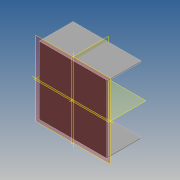
# Autodesk Inventor part: P004_CageDeTest2
Saved by Autodesk Inventor 2020 (Build 240168000, 168)
## iProperties
Created: 2021-09-24
Part Number: P004_CageDeTest2
Material: Générique
Document SubType Name: Modeling
Designer: gabri
Density: 1 g/cm^3
Appearance: Par défaut
Author: gabri
Autodesk Inventor part; units mm, degrees
sketch "Esquisse2" plane through (0, 0, 0) normal (0, 1, 0) x (-1, 0, 0)
  line L0 (1000, 1000) -> (-1000, 1000)
  line L1 (-1000, 1000) -> (-1000, -1000)
  line L2 (-1000, -1000) -> (1000, -1000)
  line L3 (1000, -1000) -> (1000, 1000)
  line L4 (0, -1400) -> (0, 1400) construction
  line L5 (1400, 0) -> (-1400, 0) construction
  point P0 (0, 0)
  dimension "d0" = 2000
  dimension "d1" = 2000
  dimension "d2" = 1000
  dimension "d3" = 1000
  constraints: 8 end point, 2 parallel, 1 horizontal, 1 perpendicular
  measures "d0" distance of L0.end L1.end
  measures "d1" distance of L0.start L0.end
  measures "d2" distance between parallel lines of L4 L1
  measures "d3" distance between parallel lines of L5 L0
extrude "Extrusion1" add sketch "Esquisse2" along normal blind 1000
sketch "Esquisse3" plane through (0, 1000, 0) normal (0, 1, 0) x (1, 0, 0)
  line L0 (-960, -960) -> (960, -960)
  line L1 (960, -960) -> (960, 960)
  line L2 (960, 960) -> (-960, 960)
  line L3 (-960, 960) -> (-960, -960)
  line L4 (1000, 1000) -> (-1000, 1000) construction
  line L5 (-1000, -1000) -> (1000, -1000) construction
  line L6 (-1000, 1000) -> (-1000, -1000) construction
  line L7 (1000, -1000) -> (1000, 1000) construction
  point P0 (0, 0)
  dimension "d6" = 40
  dimension "d7" = 40
  dimension "d8" = 40
  dimension "d9" = 40
  constraints: 8 end point, 2 parallel, 1 horizontal, 1 perpendicular
  measures "d6" distance between parallel lines of L4 L2
  measures "d7" distance between parallel lines of L5 L0
  measures "d8" distance between parallel lines of L6 L3
  measures "d9" distance between parallel lines of L7 L1
extrude "Extrusion2" cut sketch "Esquisse3" against normal blind 960
sketch "Esquisse4" plane through (1000, 0, 1000) normal (1, 0, 0) x (0, 0, -1)
  line L0 (0, 0) -> (2000, 0) construction
  line L1 (2000, 0) -> (2000, 1000) construction
  line L2 (0, 1000) -> (2000, 1000) construction
  line L3 (0, 0) -> (0, 1000) construction
  line L4 (1960, 40) -> (40, 40) construction
  line L5 (40, 1000) -> (40, 40) construction
  line L6 (1960, 1000) -> (1960, 40) construction
  line L7 (40, 1000) -> (1960, 1000)
  line L8 (1960, 1000) -> (1960, 40)
  line L9 (1960, 40) -> (40, 40)
  line L10 (40, 40) -> (40, 1000)
  point P0 (1000, 0)
  constraints: 8 end point, 2 parallel, 1 horizontal, 1 perpendicular
extrude "Extrusion3" cut sketch "Esquisse4" against normal blind 960
